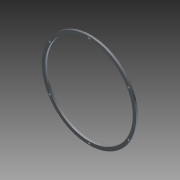
# Autodesk Inventor part: inner piece
Saved by Autodesk Inventor 2011 SP1 (Build 150282100, 282)
## iProperties
Created: 2012-01-20
Part Number: inner piece
Document SubType Name: Modeling
Designer: Christopher
Density: 1 g/cm^3
Author: Christopher
Autodesk Inventor part; units mm, degrees
ref_plane "YZ Plane" through (0, 0, 0) normal (1, 0, 0) x (0, 1, 0)
ref_plane "XZ Plane" through (0, 0, 0) normal (0, 1, 0) x (-1, 0, 0)
ref_plane "XY Plane" through (0, 0, 0) normal (0, 0, 1) x (1, 0, 0)
sketch "Sketch1" plane through (0, 0, 0) normal (0, 0, 1) x (1, 0, 0)
  circle A0 centre (0, 0) radius 142.621
  circle A1 centre (0, 0) radius 132.461
  point P0 (0, 137.541)
  point P1 (-119.114, 68.7705)
  point P2 (-119.114, -68.7705)
  point P3 (0, -137.541)
  point P4 (119.114, -68.7705)
  point P5 (119.114, 68.7705)
  dimension "d0" = 285.242
  dimension "d1" = 264.922
  dimension "d2" = 137.541
  dimension "d5" = 360
  constraints: 4 coincident, 2 centre point, 11 other
  measures "d0" diameter of A0
  measures "d1" diameter of A1
  measures "d2" distance of point (0, 137.541) A1.centre
extrude "Extrusion1" add sketch "Sketch1" against normal blind 6.096
hole "Hole1" at (0, 137.541, 0) at (-119.114, 68.7705, 0) at (-119.114, -68.7705, 0) at (0, -137.541, 0) at (119.114, -68.7705, 0) at (119.114, 68.7705, 0) direction (0, 0, -1) diameter 6.35 depth 25.4 tip angle 118
body "Solid1"
